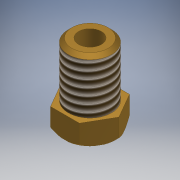
# Autodesk Inventor part: Buse 04
Saved by Autodesk Inventor 2017 (Build 210142000, 142)
## iProperties
Company: FABLAB Frenchmakers
Part Number: Buse 04
Material: Laiton, jaune doux
Document SubType Name: Modeling
Designer: FABLAB Frenchmakers
Density: 8.47 g/cm^3
Appearance: Laiton - Satiné
Mass: 2.27201 g
Surface Area: 3.91808 cm^2
Volume: 0.268242 cm^3
Project: 1420 Vauban 3D XL
Catalog Web Link: http://frenchmakers.com/
Stock Number: 1420-02-21
Autodesk Inventor part; units mm, degrees
ref_plane "YZ Plane" through (0, 0, 0) normal (1, 0, 0) x (0, 1, 0)
ref_plane "XZ Plane" through (0, 0, 0) normal (0, 1, 0) x (-1, 0, 0)
ref_plane "XY Plane" through (0, 0, 0) normal (0, 0, 1) x (1, 0, 0)
sketch "Esquisse1" plane through (0, 0, 0) normal (0, 0, 1) x (1, 0, 0)
  line L0 (2.0005, 3.465) -> (4.001, 0)
  line L1 (4.001, 0) -> (2.0005, -3.465)
  line L2 (2.0005, -3.465) -> (-2.0005, -3.465)
  line L3 (-2.0005, -3.465) -> (-4.001, 0)
  line L4 (-4.001, 0) -> (-2.0005, 3.465)
  line L5 (-2.0005, 3.465) -> (2.0005, 3.465)
  point P0 (0, 0)
  point P1 (0, 0)
  dimension "d0" = 6.93
  constraints: 12 end point, 1 coincident, 1 horizontal, 13 other
  measures "d0" distance between parallel lines of L2 L5
extrude "Extrusion1" add sketch "Esquisse1" along normal blind 3
sketch "Esquisse2" plane through (0, 0, 3) normal (0, 0, 1) x (1, 0, 0)
  circle A0 centre (0, 0) radius 3
  dimension "d3" = 6
  constraints: 1 centre point, 1 coincident
  measures "d3" diameter of A0
extrude "Extrusion2" add sketch "Esquisse2" along normal blind 7.5
sketch "Esquisse3" plane through (0, 0, 0) normal (1, 0, 0) x (0, 1, 0)
  line L0 (1.85, 0) -> (0.5, -2)
  line L1 (0.5, -2) -> (0, -2)
  line L2 (0, -2) -> (0, 0)
  line L3 (0, 0) -> (1.85, 0)
  line L4 (0, 0) -> (3.465, 0) construction
  line L5 (0, 0) -> (0, -9.9285)
  dimension "d6" = 2
  dimension "d7" = 1
  dimension "d8" = 3.7
  constraints: 10 end point, 1 collinear, 1 horizontal, 1 perpendicular, 1 vertical
  measures "d6" distance between parallel lines of L4 L1
  measures "d7" diameter of L0.end L5
  measures "d8" diameter of L0.start L5
revolve "Révolution1" add sketch "Esquisse3" angle 360 about axis through (0, 0, 0) along (0, 0, -1)
chamfer "Chanfrein1" distance 0.5 angle 45 1 edges at (-3, 0, 10.5)
thread "Filetage1" size "M6x1" class "6g" standard "ANSI Metric M Profile" full length
sketch "Esquisse4" plane through (0, 0, 0) normal (0, 1, 0) x (-1, 0, 0)
  line L0 (2.0005, 0) -> (4.001, 0) projected
  line L1 (3.501, 0) -> (4.001, 0.5)
  line L2 (4.001, 0.5) -> (4.001, 0)
  line L3 (4.001, 0) -> (3.501, 0)
  line L4 (0, 0) -> (0, 3.501)
  dimension "d15" = 0.5
  dimension "d16" = 0.5
  constraints: 8 end point, 3 point on line, 1 perpendicular, 1 vertical
  measures "d15" distance of L1.end L0.end
  measures "d16" distance from line of L2 L1.start
revolve "Révolution2" cut sketch "Esquisse4" angle 360 about axis through (0, 0, 0) along (0, 0, 1)
fillet "Congé1" radius 0.5 1 edges at (0, -1.85, 0)
sketch "Esquisse5" plane through (0, 0, 10.5) normal (0, 0, 1) x (1, 0, 0)
  point P0 (0, 0)
  point P1 (0, 0)
  constraints: 1 coincident
hole "Perçage1" at (0, 0, 10.5) direction (0, 0, -1) diameter 0.4 end through all counterbore diameter 3.15 counterbore depth 10.5
sketch "Esquisse6" plane through (-2.0005, 3.465, 3) normal (0, 1, 0) x (1, 0, 0)
  line L0 (1.4995, 3) -> (2.5016, 3) construction
  line L1 (4.7508, 3) -> (2.5016, 3) construction
  line L2 (6.0016, 0) -> (4.001, 0) construction
  point P0 (2.0005, 3)
  point P1 (2.0005, 1.5)
  point P2 (4.001, 1.5)
  point P3 (2.0005, 3)
  dimension "d26" = 3
  dimension "d27" = 1.5
  constraints: 1 horizontal alignment, 1 midpoint, 1 vertical alignment
  measures "d26" distance between parallel lines of L2 L1
  measures "d27" distance from line of L2 point (2.001, 1.5)
hole "Perçage2" at (0, 3.465, 1.5) direction (0, -1, 0) diameter 1 depth 0.01 tip angle 118
pattern_circular "Réseau circulaire1" count 2 over 60 about axis through (0, 0, -5.8801) along (0, 0, 1) of "Perçage2"
chamfer "Chanfrein2" distance 1.375 angle 45 1 edges at (0, 1.575, 0)
equation "\"d16\" = d15"
equation "\"d27\" = 0.5 * d26"
